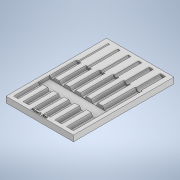
# Autodesk Inventor part: punchTray
Saved by Autodesk Inventor 2020.2 (Build 242310000, 310)
## iProperties
Created: 2019-12-07
Part Number: punchTray
Material: Generic
Document SubType Name: Modeling
Designer: robst
Density: 1 g/cm^3
Appearance: Default
Author: robst
Autodesk Inventor part; units mm, degrees
(part 1 of 2)
ref_plane "YZ Plane" through (0, 0, 0) normal (1, 0, 0) x (0, 1, 0)
ref_plane "XZ Plane" through (0, 0, 0) normal (0, 1, 0) x (-1, 0, 0)
ref_plane "XY Plane" through (0, 0, 0) normal (0, 0, 1) x (1, 0, 0)
sketch "Sketch3" plane through (0, 0, 0) normal (0, 0, 1) x (1, 0, 0)
  line L0 (-56.4324, -4.8895) -> (56.4324, -4.8895)
  line L1 (56.4324, -4.8895) -> (56.4324, 4.8895)
  line L2 (56.4324, 4.8895) -> (-56.4324, 4.8895)
  line L3 (-56.4324, 4.8895) -> (-56.4324, -4.8895)
  line L4 (-56.4324, -4.8895) -> (56.4324, 4.8895) construction
  line L5 (56.4324, -4.8895) -> (-56.4324, 4.8895) construction
  line L6 (50.0824, 4.8895) -> (47.1861, -0.127)
  line L7 (47.1861, -0.127) -> (41.3935, -0.127)
  line L8 (41.3935, -0.127) -> (38.4972, 4.8895)
  line L9 (38.4972, 4.8895) -> (41.3935, 9.906)
  line L10 (41.3935, 9.906) -> (47.1861, 9.906)
  line L11 (47.1861, 9.906) -> (50.0824, 4.8895)
  line L12 (30.5597, 4.8895) -> (27.6635, -0.127)
  line L13 (27.6635, -0.127) -> (21.8709, -0.127)
  line L14 (21.8709, -0.127) -> (18.9746, 4.8895)
  line L15 (18.9746, 4.8895) -> (21.8709, 9.906)
  line L16 (21.8709, 9.906) -> (27.6635, 9.906)
  line L17 (27.6635, 9.906) -> (30.5597, 4.8895)
  line L18 (0, 0) -> (0, 4.8895) construction
  line L19 (11.0371, 4.8895) -> (8.5808, 0.635)
  line L20 (8.5808, 0.635) -> (3.6681, 0.635)
  line L21 (3.6681, 0.635) -> (1.2118, 4.8895)
  line L22 (1.2118, 4.8895) -> (3.6681, 9.144)
  line L23 (3.6681, 9.144) -> (8.5808, 9.144)
  line L24 (8.5808, 9.144) -> (11.0371, 4.8895)
  line L25 (-6.7257, 4.8895) -> (-9.182, 0.635)
  line L26 (-9.182, 0.635) -> (-14.0947, 0.635)
  line L27 (-14.0947, 0.635) -> (-16.5511, 4.8895)
  line L28 (-16.5511, 4.8895) -> (-14.0947, 9.144)
  line L29 (-14.0947, 9.144) -> (-9.182, 9.144)
  line L30 (-9.182, 9.144) -> (-6.7257, 4.8895)
  line L31 (-24.4886, 4.8895) -> (-26.9229, 0.6731)
  line L32 (-26.9229, 0.6731) -> (-31.7916, 0.6731)
  line L33 (-31.7916, 0.6731) -> (-34.2259, 4.8895)
  line L34 (-34.2259, 4.8895) -> (-31.7916, 9.1059)
  line L35 (-31.7916, 9.1059) -> (-26.9229, 9.1059)
  line L36 (-26.9229, 9.1059) -> (-24.4886, 4.8895)
  line L37 (-42.1634, 4.8895) -> (-44.1432, 1.4605)
  line L38 (-44.1432, 1.4605) -> (-48.1026, 1.4605)
  line L39 (-48.1026, 1.4605) -> (-50.0824, 4.8895)
  line L40 (-50.0824, 4.8895) -> (-48.1026, 8.3185)
  line L41 (-48.1026, 8.3185) -> (-44.1432, 8.3185)
  line L42 (-44.1432, 8.3185) -> (-42.1634, 4.8895)
  point P0 (44.2898, 4.8895)
  point P1 (24.7672, 4.8895)
  point P2 (38.4972, 4.8895)
  point P3 (18.9746, 4.8895)
  point P4 (6.1245, 4.8895)
  point P5 (-11.6384, 4.8895)
  point P6 (-29.3572, 4.8895)
  point P7 (-46.1229, 4.8895)
  point P8 (1.2118, 4.8895)
  point P9 (-16.5511, 4.8895)
  point P10 (-34.2259, 4.8895)
  point P11 (-50.0824, 4.8895)
  dimension "d7" = 10.033
  dimension "d8" = 10.033
  dimension "d13" = 6.35
  dimension "d14" = 7.9375
  dimension "d15" = 8.509
  dimension "d16" = 7.9375
  dimension "d17" = 8.509
  dimension "d18" = 7.9375
  dimension "d19" = 8.4328
  dimension "d20" = 7.9375
  dimension "d21" = 7.9375
  dimension "d22" = 6.858
  dimension "d23" = 6.35
  dimension "d24" = 4.7625
  constraints: 84 end point, 2 horizontal, 2 midpoint, 1 parallel, 1 perpendicular, 94 other
  measures "d7" distance between parallel lines of L7 L10
  measures "d8" distance between parallel lines of L13 L16
  measures "d13" distance of L6.start L1.end
  measures "d14" distance of L8.end L12.start
  measures "d15" distance between parallel lines of L20 L23
  measures "d16" distance of L14.end L19.start
  measures "d17" distance between parallel lines of L26 L29
  measures "d18" distance of L21.end L25.start
  measures "d19" distance between parallel lines of L32 L35
  measures "d20" distance of L27.end L31.start
  measures "d21" distance of L33.end L37.start
  measures "d22" distance between parallel lines of L38 L41
  measures "d23" distance from line of L39.end L3
  measures "d24" distance between parallel lines of L0 L7
extrude "Extrusion3" add sketch "Sketch3" against normal blind 155.575 contours L3 L2 L39 L38 L37 L33 L32 L31 L27 L26 L25 L21 L20 L19 L14 L13 L12 L8 L7 L6 L1 L0
sketch "Sketch4" plane through (0, 0, 0) normal (0, 0, 1) x (1, 0, 0)
  line L0 (56.4324, -4.8895) -> (-56.4324, -4.8895) projected
  line L1 (56.4324, 4.8895) -> (56.4324, -4.8895) projected
  line L2 (-56.4324, -4.8895) -> (56.4324, -4.8895)
  line L3 (56.4324, -4.8895) -> (56.4324, 4.8895)
  line L4 (56.4324, 4.8895) -> (-56.4324, 4.8895)
  line L5 (-56.4324, 4.8895) -> (-56.4324, -4.8895)
  point P0 (0, 0)
  constraints: 8 end point, 2 parallel, 1 horizontal, 1 perpendicular
extrude "Extrusion4" add sketch "Sketch4" along normal blind 6.35
sketch "Sketch6" plane through (0, 0, -155.575) normal (0, 0, -1) x (-1, 0, 0)
  line L0 (-41.3935, -0.127) -> (-47.1861, -0.127) construction
  line L1 (-44.2898, -0.127) -> (-44.2898, 4.8895) construction
  line L2 (-56.4324, 4.8895) -> (56.4324, 4.8895) construction
  arc A0 (-48.5125, 4.8895) -> (-40.067, 4.8895) centre (-44.2898, 4.8895) ccw
  line L3 (-38.4972, 4.8895) -> (-41.3935, -0.127)
  line L4 (-41.3935, -0.127) -> (-47.1861, -0.127)
  line L5 (-47.1861, -0.127) -> (-50.0824, 4.8895)
  line L6 (-50.0824, 4.8895) -> (-48.5125, 4.8895)
  line L7 (-38.4972, 4.8895) -> (-40.067, 4.8895)
  point P0 (0, 0)
  dimension "d31" = 8.4455
  constraints: 12 end point, 3 point on line, 2 coincident, 2 point on circle, 1 centre point, 1 midpoint, 1 vertical, 6 other
  measures "d31" diameter of A0
extrude "5_16_punch" add sketch "Sketch6" against normal blind 40.64
sketch "Sketch7" plane through (0, 0, -155.575) normal (0, 0, -1) x (-1, 0, 0)
  line L0 (-30.5597, 4.8895) -> (-18.9746, 4.8895) projected
  line L1 (-18.9746, 4.8895) -> (-21.8709, -0.127)
  line L2 (-21.8709, -0.127) -> (-27.6635, -0.127)
  line L3 (-27.6635, -0.127) -> (-30.5597, 4.8895)
  arc A0 (-28.1962, 4.8895) -> (-21.3382, 4.8895) centre (-24.7672, 4.8895) ccw
  line L4 (-30.5597, 4.8895) -> (-28.1962, 4.8895)
  line L5 (-11.0371, 4.8895) -> (-18.9746, 4.8895) projected
  line L6 (-18.9746, 4.8895) -> (-21.3382, 4.8895)
  point P0 (0, 0)
  point P1 (-30.5597, 4.8895)
  dimension "d34" = 6.858
  constraints: 10 end point, 2 point on circle, 2 point on line, 1 centre point, 1 coincident, 1 midpoint, 6 other
  measures "d34" diameter of A0
extrude "1_4_punch" add sketch "Sketch7" against normal blind 40.64 contours L0 A0 L1 L2 L3
sketch "Sketch8" plane through (0, 0, -155.575) normal (0, 0, -1) x (-1, 0, 0)
  line L0 (-11.0371, 4.8895) -> (-1.2118, 4.8895) projected
  line L1 (-1.2118, 4.8895) -> (-3.6681, 0.635)
  line L2 (-3.6681, 0.635) -> (-8.5808, 0.635)
  line L3 (-8.5808, 0.635) -> (-11.0371, 4.8895)
  arc A0 (-8.7597, 4.8895) -> (-3.4892, 4.8895) centre (-6.1245, 4.8895) ccw
  line L4 (-11.0371, 4.8895) -> (-8.5808, 0.635) projected
  line L5 (-11.0371, 4.8895) -> (-8.7597, 4.8895)
  line L6 (-1.2118, 4.8895) -> (-3.4892, 4.8895)
  point P0 (0, 0)
  point P1 (-11.0371, 4.8895)
  dimension "d37" = 5.2705
  constraints: 10 end point, 2 point on circle, 2 point on line, 1 centre point, 1 coincident, 1 midpoint, 6 other
  measures "d37" diameter of A0
extrude "3_16_punch" add sketch "Sketch8" against normal blind 40.64 contours L0 A0 L1 L2 L3
sketch "Sketch9" plane through (0, 0, -155.575) normal (0, 0, -1) x (-1, 0, 0)
  line L0 (14.0947, 0.635) -> (9.182, 0.635) construction
  line L1 (11.6384, 0.635) -> (11.6384, 4.8895) construction
  line L2 (-56.4324, 4.8895) -> (56.4324, 4.8895) construction
  line L3 (16.5511, 4.8895) -> (14.0947, 0.635) projected
  line L4 (16.5511, 4.8895) -> (14.0947, 0.635)
  line L5 (14.0947, 0.635) -> (9.182, 0.635)
  line L6 (9.182, 0.635) -> (6.7257, 4.8895)
  arc A0 (9.4, 4.8895) -> (13.8768, 4.8895) centre (11.6384, 4.8895) ccw
  line L7 (9.182, 0.635) -> (6.7257, 4.8895) projected
  line L8 (6.7257, 4.8895) -> (9.4, 4.8895)
  line L9 (24.4886, 4.8895) -> (16.5511, 4.8895) projected
  line L10 (16.5511, 4.8895) -> (13.8768, 4.8895)
  point P0 (0, 0)
  point P1 (14.0947, 0.635)
  dimension "d40" = 4.4768
  constraints: 12 end point, 3 point on line, 2 coincident, 2 point on circle, 1 centre point, 1 midpoint, 1 vertical, 6 other
  measures "d40" diameter of A0
extrude "5_32_punch" add sketch "Sketch9" against normal blind 45.72
sketch "Sketch11" plane through (0, 0, -155.575) normal (0, 0, -1) x (-1, 0, 0)
  line L0 (24.4886, 4.8895) -> (34.2259, 4.8895) projected
  line L1 (31.7916, 0.6731) -> (34.2259, 4.8895) projected
  line L2 (34.2259, 4.8895) -> (31.7916, 0.6731)
  line L3 (31.7916, 0.6731) -> (26.9229, 0.6731)
  line L4 (26.9229, 0.6731) -> (24.4886, 4.8895)
  arc A0 (27.5157, 4.8895) -> (31.1987, 4.8895) centre (29.3572, 4.8895) ccw
  line L5 (24.4886, 4.8895) -> (26.9229, 0.6731) projected
  line L6 (24.4886, 4.8895) -> (27.5157, 4.8895)
  line L7 (34.2259, 4.8895) -> (31.1987, 4.8895)
  point P0 (0, 0)
  point P1 (31.7916, 0.6731)
  point P2 (24.4886, 4.8895)
  dimension "d44" = 3.683
  constraints: 10 end point, 2 point on circle, 2 point on line, 1 centre point, 1 coincident, 1 midpoint, 6 other
  measures "d44" diameter of A0
extrude "1_8_punch" add sketch "Sketch11" against normal blind 50.8 contours L0 A0 L1 L3 L4
sketch "Sketch12" plane through (0, 0, -155.575) normal (0, 0, -1) x (-1, 0, 0)
  line L0 (44.1432, 1.4605) -> (48.1026, 1.4605) construction
  line L1 (46.1229, 1.4605) -> (46.1229, 4.8895) construction
  line L2 (-56.4324, 4.8895) -> (56.4324, 4.8895) construction
  line L3 (48.1026, 1.4605) -> (50.0824, 4.8895) projected
  line L4 (50.0824, 4.8895) -> (48.1026, 1.4605)
  line L5 (48.1026, 1.4605) -> (44.1432, 1.4605)
  line L6 (44.1432, 1.4605) -> (42.1634, 4.8895)
  arc A0 (45.0751, 4.8895) -> (47.1706, 4.8895) centre (46.1229, 4.8895) ccw
  line L7 (42.1634, 4.8895) -> (31.1987, 4.8895) projected
  line L8 (42.1634, 4.8895) -> (45.0751, 4.8895)
  line L9 (50.0824, 4.8895) -> (47.1706, 4.8895)
  point P0 (0, 0)
  dimension "d47" = 2.0955
  constraints: 12 end point, 3 point on line, 2 coincident, 2 point on circle, 1 centre point, 1 midpoint, 1 vertical, 6 other
  measures "d47" diameter of A0
extrude "1_16_punch" add sketch "Sketch12" against normal blind 50.8
sketch "Sketch5" plane through (0, 0, -155.575) normal (0, 0, -1) x (-1, 0, 0)
  line L0 (-56.4324, 4.8895) -> (-56.4324, -4.8895) projected
  line L1 (56.4324, 4.8895) -> (50.0824, 4.8895) projected
  line L2 (-56.4324, -4.8895) -> (56.4324, -4.8895)
  line L3 (56.4324, -4.8895) -> (56.4324, 4.8895)
  line L4 (56.4324, 4.8895) -> (-56.4324, 4.8895)
  line L5 (-56.4324, 4.8895) -> (-56.4324, -4.8895)
  point P0 (0, 0)
  point P1 (-56.4324, 4.8895)
  constraints: 8 end point, 2 parallel, 1 horizontal, 1 perpendicular
extrude "Extrusion5" add sketch "Sketch5" along normal blind 6.35
sketch "Sketch13" plane through (-56.4324, 4.8895, 6.35) normal (0, 1, 0) x (1, 0, 0)
  line L0 (6.35, 6.35) -> (6.35, 111.125) projected
  line L1 (106.5147, 6.35) -> (106.5147, 121.285) projected
  line L2 (6.35, 47.625) -> (106.5147, 47.625)
  line L3 (106.5147, 47.625) -> (106.5147, 66.675)
  line L4 (106.5147, 66.675) -> (6.35, 66.675)
  line L5 (6.35, 66.675) -> (6.35, 47.625)
  line L6 (6.35, 57.15) -> (106.5147, 57.15) construction
  line L7 (14.2689, 6.35) -> (6.35, 6.35) construction
  point P0 (56.4324, 6.35)
  point P1 (6.35, 66.675)
  point P2 (106.5147, 47.625)
  dimension "d50" = 19.05
  dimension "d51" = 50.8
  constraints: 10 end point, 2 midpoint, 2 parallel, 2 point on line, 1 horizontal, 1 perpendicular
  measures "d50" distance between parallel lines of L4 L2
  measures "d51" distance between parallel lines of L6 L7
extrude "Extrusion12" cut sketch "Sketch13" against normal blind 5.08
sketch "Sketch14" plane through (-56.4324, 4.8895, 6.35) normal (0, 1, 0) x (1, 0, 0)
  line L0 (0, 168.275) -> (0, 0) construction
  line L1 (0, 3.175) -> (104.9272, 3.175) construction
  line L2 (0, 0) -> (112.8647, 0) construction
  spline S0 degree 2 poles (42.5851, 3.879) (42.5851, 3.6134) (42.4153, 3.1318) (42.2578, 2.9712) knots 0 0 0 1 2 2 2
  spline S1 degree 2 poles (42.2578, 2.9712) (42.1621, 2.8693) (41.9274, 2.7026) (41.7885, 2.6439) knots 0 0 0 1 2 2 2
  spline S2 degree 2 poles (41.7885, 2.6439) (41.6465, 2.5853) (41.3161, 2.5174) (41.1123, 2.5174) knots 0 0 0 1 2 2 2
  line L3 (41.1123, 2.5174) -> (40.6122, 2.5174)
  line L4 (40.6122, 2.5174) -> (40.6122, 1.27)
  line L5 (40.6122, 1.27) -> (39.655, 1.27)
  line L6 (39.655, 1.27) -> (39.655, 5.08)
  line L7 (39.655, 5.08) -> (41.1339, 5.08)
  spline S3 degree 2 poles (41.1339, 5.08) (41.4612, 5.08) (41.9398, 4.9596) (42.1343, 4.8299) knots 0 0 0 1 2 2 2
  spline S4 degree 2 poles (42.1343, 4.8299) (42.3504, 4.6848) (42.5851, 4.2093) (42.5851, 3.879) knots 0 0 0 1 2 2 2
  spline S5 degree 2 poles (41.6033, 3.8543) (41.6033, 4.0179) (41.4489, 4.2495) (41.3439, 4.2927) knots 0 0 0 1 2 2 2
  spline S6 degree 2 poles (41.3439, 4.2927) (41.208, 4.3513) (40.961, 4.3699) (40.748, 4.3699) knots 0 0 0 1 2 2 2
  line L8 (40.748, 4.3699) -> (40.6122, 4.3699)
  line L9 (40.6122, 4.3699) -> (40.6122, 3.2275)
  line L10 (40.6122, 3.2275) -> (40.6801, 3.2275)
  spline S7 degree 2 poles (40.6801, 3.2275) (40.8128, 3.2275) (41.0537, 3.2337) (41.1432, 3.2491) knots 0 0 0 1 2 2 2
  spline S8 degree 2 poles (41.1432, 3.2491) (41.2204, 3.2615) (41.3902, 3.3356) (41.4365, 3.3819) knots 0 0 0 1 2 2 2
  spline S9 degree 2 poles (41.4365, 3.3819) (41.5353, 3.4745) (41.6033, 3.6814) (41.6033, 3.8543) knots 0 0 0 1 2 2 2
  line L11 (45.7127, 1.27) -> (44.8174, 1.27)
  line L12 (44.8174, 1.27) -> (44.8174, 1.588)
  spline S10 degree 2 poles (44.8174, 1.588) (44.5858, 1.3935) (44.1968, 1.1897) (43.9282, 1.1897) knots 0 0 0 1 2 2 2
  spline S11 degree 2 poles (43.9282, 1.1897) (43.5021, 1.1897) (43.0235, 1.73) (43.0235, 2.2734) knots 0 0 0 1 2 2 2
  line L13 (43.0235, 2.2734) -> (43.0235, 4.1445)
  line L14 (43.0235, 4.1445) -> (43.9251, 4.1445)
  line L15 (43.9251, 4.1445) -> (43.9251, 2.718)
  spline S12 degree 2 poles (43.9251, 2.718) (43.9251, 2.4957) (43.9467, 2.2117) (43.9899, 2.116) knots 0 0 0 1 2 2 2
  spline S13 degree 2 poles (43.9899, 2.116) (44.0331, 2.0264) (44.2029, 1.9338) (44.3573, 1.9338) knots 0 0 0 1 2 2 2
  spline S14 degree 2 poles (44.3573, 1.9338) (44.4499, 1.9338) (44.7093, 2.0264) (44.8174, 2.1067) knots 0 0 0 1 2 2 2
  line L16 (44.8174, 2.1067) -> (44.8174, 4.1445)
  line L17 (44.8174, 4.1445) -> (45.7127, 4.1445)
  line L18 (45.7127, 4.1445) -> (45.7127, 1.27)
  line L19 (49.0874, 1.27) -> (48.1858, 1.27)
  line L20 (48.1858, 1.27) -> (48.1858, 2.6933)
  spline S15 degree 2 poles (48.1858, 2.6933) (48.1858, 2.8693) (48.1581, 3.2151) (48.121, 3.2954) knots 0 0 0 1 2 2 2
  spline S16 degree 2 poles (48.121, 3.2954) (48.0747, 3.3942) (47.9018, 3.4776) (47.7536, 3.4776) knots 0 0 0 1 2 2 2
  spline S17 degree 2 poles (47.7536, 3.4776) (47.6455, 3.4776) (47.4201, 3.3942) (47.2936, 3.3047) knots 0 0 0 1 2 2 2
  line L21 (47.2936, 3.3047) -> (47.2936, 1.27)
  line L22 (47.2936, 1.27) -> (46.3982, 1.27)
  line L23 (46.3982, 1.27) -> (46.3982, 4.1445)
  line L24 (46.3982, 4.1445) -> (47.2936, 4.1445)
  line L25 (47.2936, 4.1445) -> (47.2936, 3.8265)
  spline S18 degree 2 poles (47.2936, 3.8265) (47.5128, 4.0117) (47.9296, 4.2217) (48.1828, 4.2217) knots 0 0 0 1 2 2 2
  spline S19 degree 2 poles (48.1828, 4.2217) (48.6212, 4.2217) (49.0874, 3.6659) (49.0874, 3.141) knots 0 0 0 1 2 2 2
  line L26 (49.0874, 3.141) -> (49.0874, 1.27)
  spline S20 degree 2 poles (51.1591, 1.1928) (50.8041, 1.1928) (50.2143, 1.3719) (49.9951, 1.5571) knots 0 0 0 1 2 2 2
  spline S21 degree 2 poles (49.9951, 1.5571) (49.7821, 1.7455) (49.5413, 2.3105) (49.5413, 2.6933) knots 0 0 0 1 2 2 2
  spline S22 degree 2 poles (49.5413, 2.6933) (49.5413, 3.1071) (49.8006, 3.6844) (50.026, 3.8697) knots 0 0 0 1 2 2 2
  spline S23 degree 2 poles (50.026, 3.8697) (50.239, 4.0488) (50.8195, 4.2217) (51.1344, 4.2217) knots 0 0 0 1 2 2 2
  spline S24 degree 2 poles (51.1344, 4.2217) (51.3722, 4.2217) (51.8476, 4.1105) (52.0885, 3.9901) knots 0 0 0 1 2 2 2
  line L27 (52.0885, 3.9901) -> (52.0885, 3.2244)
  line L28 (52.0885, 3.2244) -> (51.9742, 3.2244)
  spline S25 degree 2 poles (51.9742, 3.2244) (51.9187, 3.2769) (51.7643, 3.4004) (51.6717, 3.4498) knots 0 0 0 1 2 2 2
  spline S26 degree 2 poles (51.6717, 3.4498) (51.5729, 3.5054) (51.3289, 3.5795) (51.1777, 3.5795) knots 0 0 0 1 2 2 2
  spline S27 degree 2 poles (51.1777, 3.5795) (50.8349, 3.5795) (50.4583, 3.1009) (50.4583, 2.6933) knots 0 0 0 1 2 2 2
  spline S28 degree 2 poles (50.4583, 2.6933) (50.4583, 2.2611) (50.8596, 1.835) (51.1931, 1.835) knots 0 0 0 1 2 2 2
  spline S29 degree 2 poles (51.1931, 1.835) (51.3629, 1.835) (51.6161, 1.9122) (51.7087, 1.9678) knots 0 0 0 1 2 2 2
  spline S30 degree 2 poles (51.7087, 1.9678) (51.7982, 2.0203) (51.9279, 2.1376) (51.9742, 2.1839) knots 0 0 0 1 2 2 2
  line L29 (51.9742, 2.1839) -> (52.0885, 2.1839)
  line L30 (52.0885, 2.1839) -> (52.0885, 1.4151)
  spline S31 degree 2 poles (52.0885, 1.4151) (52.0113, 1.3812) (51.8106, 1.2947) (51.7056, 1.2669) knots 0 0 0 1 2 2 2
  spline S32 degree 2 poles (51.7056, 1.2669) (51.5759, 1.2299) (51.3475, 1.1928) (51.1591, 1.1928) knots 0 0 0 1 2 2 2
  line L31 (55.2038, 1.27) -> (54.3022, 1.27)
  line L32 (54.3022, 1.27) -> (54.3022, 2.6933)
  spline S33 degree 2 poles (54.3022, 2.6933) (54.3022, 2.8693) (54.2744, 3.2151) (54.2374, 3.2954) knots 0 0 0 1 2 2 2
  spline S34 degree 2 poles (54.2374, 3.2954) (54.1911, 3.3942) (54.0182, 3.4776) (53.87, 3.4776) knots 0 0 0 1 2 2 2
  spline S35 degree 2 poles (53.87, 3.4776) (53.7619, 3.4776) (53.5365, 3.3942) (53.4099, 3.3047) knots 0 0 0 1 2 2 2
  line L33 (53.4099, 3.3047) -> (53.4099, 1.27)
  line L34 (53.4099, 1.27) -> (52.5145, 1.27)
  line L35 (52.5145, 1.27) -> (52.5145, 5.2498)
  line L36 (52.5145, 5.2498) -> (53.4099, 5.2498)
  line L37 (53.4099, 5.2498) -> (53.4099, 3.8265)
  spline S36 degree 2 poles (53.4099, 3.8265) (53.6291, 4.0117) (54.046, 4.2217) (54.2991, 4.2217) knots 0 0 0 1 2 2 2
  spline S37 degree 2 poles (54.2991, 4.2217) (54.7376, 4.2217) (55.2038, 3.6659) (55.2038, 3.141) knots 0 0 0 1 2 2 2
  line L38 (55.2038, 3.141) -> (55.2038, 1.27)
  spline S38 degree 2 poles (58.6309, 1.2021) (58.1925, 1.2021) (57.5318, 1.3719) (57.2477, 1.4954) knots 0 0 0 1 2 2 2
  line L39 (57.2477, 1.4954) -> (57.2477, 2.4031)
  line L40 (57.2477, 2.4031) -> (57.3342, 2.4031)
  spline S39 degree 2 poles (57.3342, 2.4031) (57.6213, 2.1592) (58.3098, 1.8968) (58.634, 1.8968) knots 0 0 0 1 2 2 2
  spline S40 degree 2 poles (58.634, 1.8968) (58.7174, 1.8968) (58.986, 1.9338) (59.0663, 1.9709) knots 0 0 0 1 2 2 2
  spline S41 degree 2 poles (59.0663, 1.9709) (59.1651, 2.0141) (59.304, 2.1716) (59.304, 2.2981) knots 0 0 0 1 2 2 2
  spline S42 degree 2 poles (59.304, 2.2981) (59.304, 2.4433) (59.0786, 2.6223) (58.9242, 2.6625) knots 0 0 0 1 2 2 2
  spline S43 degree 2 poles (58.9242, 2.6625) (58.7297, 2.715) (58.2882, 2.8045) (58.0937, 2.8724) knots 0 0 0 1 2 2 2
  spline S44 degree 2 poles (58.0937, 2.8724) (57.6522, 3.0268) (57.2693, 3.5548) (57.2693, 3.95) knots 0 0 0 1 2 2 2
  spline S45 degree 2 poles (57.2693, 3.95) (57.2693, 4.4841) (58.174, 5.1479) (58.8532, 5.1479) knots 0 0 0 1 2 2 2
  spline S46 degree 2 poles (58.8532, 5.1479) (59.1929, 5.1479) (59.8659, 5.009) (60.1315, 4.8917) knots 0 0 0 1 2 2 2
  line L41 (60.1315, 4.8917) -> (60.1315, 4.021)
  line L42 (60.1315, 4.021) -> (60.0481, 4.021)
  spline S47 degree 2 poles (60.0481, 4.021) (59.8351, 4.2031) (59.2237, 4.4532) (58.9026, 4.4532) knots 0 0 0 1 2 2 2
  spline S48 degree 2 poles (58.9026, 4.4532) (58.776, 4.4532) (58.5784, 4.4162) (58.4673, 4.3668) knots 0 0 0 1 2 2 2
  spline S49 degree 2 poles (58.4673, 4.3668) (58.3778, 4.3266) (58.2481, 4.1661) (58.2481, 4.0673) knots 0 0 0 1 2 2 2
  spline S50 degree 2 poles (58.2481, 4.0673) (58.2481, 3.9191) (58.4549, 3.7493) (58.7513, 3.6814) knots 0 0 0 1 2 2 2
  spline S51 degree 2 poles (58.7513, 3.6814) (58.9428, 3.6381) (59.2978, 3.5548) (59.5016, 3.4838) knots 0 0 0 1 2 2 2
  spline S52 degree 2 poles (59.5016, 3.4838) (59.8968, 3.3386) (60.2828, 2.857) (60.2828, 2.4618) knots 0 0 0 1 2 2 2
  spline S53 degree 2 poles (60.2828, 2.4618) (60.2828, 1.8937) (59.3905, 1.2021) (58.6309, 1.2021) knots 0 0 0 1 2 2 2
  spline S54 degree 2 poles (62.1939, 1.1928) (61.3788, 1.1928) (60.5112, 1.9709) (60.5112, 2.6903) knots 0 0 0 1 2 2 2
  spline S55 degree 2 poles (60.5112, 2.6903) (60.5112, 3.3942) (61.3202, 4.234) (62.0488, 4.234) knots 0 0 0 1 2 2 2
  spline S56 degree 2 poles (62.0488, 4.234) (62.7065, 4.234) (63.3734, 3.5208) (63.3734, 2.8601) knots 0 0 0 1 2 2 2
  line L43 (63.3734, 2.8601) -> (63.3734, 2.5359)
  line L44 (63.3734, 2.5359) -> (61.4066, 2.5359)
  spline S57 degree 2 poles (61.4066, 2.5359) (61.419, 2.3352) (61.5641, 2.0697) (61.6814, 1.9894) knots 0 0 0 1 2 2 2
  spline S58 degree 2 poles (61.6814, 1.9894) (61.7956, 1.9091) (62.1044, 1.8412) (62.2866, 1.8412) knots 0 0 0 1 2 2 2
  spline S59 degree 2 poles (62.2866, 1.8412) (62.4409, 1.8412) (62.7435, 1.9091) (62.8701, 1.9678) knots 0 0 0 1 2 2 2
  spline S60 degree 2 poles (62.8701, 1.9678) (62.9812, 2.0141) (63.1665, 2.1283) (63.2252, 2.1716) knots 0 0 0 1 2 2 2
  line L45 (63.2252, 2.1716) -> (63.3209, 2.1716)
  line L46 (63.3209, 2.1716) -> (63.3209, 1.4306)
  spline S61 degree 2 poles (63.3209, 1.4306) (63.2097, 1.3873) (63.0306, 1.3132) (62.8701, 1.2762) knots 0 0 0 1 2 2 2
  spline S62 degree 2 poles (62.8701, 1.2762) (62.725, 1.236) (62.4162, 1.1928) (62.1939, 1.1928) knots 0 0 0 1 2 2 2
  spline S63 degree 2 poles (62.4903, 3.0762) (62.4842, 3.3603) (62.2341, 3.6597) (61.9778, 3.6597) knots 0 0 0 1 2 2 2
  spline S64 degree 2 poles (61.9778, 3.6597) (61.7154, 3.6597) (61.419, 3.3448) (61.4035, 3.0762) knots 0 0 0 1 2 2 2
  line L47 (61.4035, 3.0762) -> (62.4903, 3.0762)
  spline S65 degree 2 poles (64.9326, 1.2144) (64.3861, 1.2144) (63.8859, 1.6652) (63.8859, 2.1777) knots 0 0 0 1 2 2 2
  line L48 (63.8859, 2.1777) -> (63.8859, 3.5208)
  line L49 (63.8859, 3.5208) -> (63.5432, 3.5208)
  line L50 (63.5432, 3.5208) -> (63.5432, 4.1445)
  line L51 (63.5432, 4.1445) -> (63.8859, 4.1445)
  line L52 (63.8859, 4.1445) -> (63.8859, 4.9658)
  line L53 (63.8859, 4.9658) -> (64.7813, 4.9658)
  line L54 (64.7813, 4.9658) -> (64.7813, 4.1445)
  line L55 (64.7813, 4.1445) -> (65.6458, 4.1445)
  line L56 (65.6458, 4.1445) -> (65.6458, 3.5208)
  line L57 (65.6458, 3.5208) -> (64.7813, 3.5208)
  line L58 (64.7813, 3.5208) -> (64.7813, 2.4988)
  spline S66 degree 2 poles (64.7813, 2.4988) (64.7813, 2.3475) (64.7874, 2.1222) (64.8245, 2.0326) knots 0 0 0 1 2 2 2
  spline S67 degree 2 poles (64.8245, 2.0326) (64.8615, 1.9431) (65.0437, 1.8381) (65.2166, 1.8381) knots 0 0 0 1 2 2 2
  spline S68 degree 2 poles (65.2166, 1.8381) (65.2907, 1.8381) (65.5223, 1.8999) (65.5686, 1.9246) knots 0 0 0 1 2 2 2
  line L59 (65.5686, 1.9246) -> (65.6458, 1.9246)
  line L60 (65.6458, 1.9246) -> (65.6458, 1.2947)
  spline S69 degree 2 poles (65.6458, 1.2947) (65.5007, 1.2576) (65.1734, 1.2144) (64.9326, 1.2144) knots 0 0 0 1 2 2 2
  point P0 (56.4324, 6.35)
  dimension "d54" = 3.175
  constraints: 2 end point, 1 horizontal, 1 parallel, 1 point on line
  measures "d54" distance between parallel lines of L1 L2
extrude "Extrusion13" cut sketch "Sketch14" against normal blind 3.175
sketch "Sketch15" plane through (-56.4324, -4.8895, 6.35) normal (0, -1, 0) x (1, 0, 0)
  line L0 (112.8647, -168.275) -> (112.8647, 0) construction
  line L1 (112.8647, -84.1375) -> (0, -84.1375) construction
  line L2 (0, -168.275) -> (0, 0) construction
  spline S0 degree 2 poles (77.0158, -94.2924) (77.0158, -93.4021) (77.7928, -92.0024) (78.3846, -91.6268) knots 0 0 0 1 2 2 2
  spline S1 degree 2 poles (78.3846, -91.6268) (78.8786, -91.3078) (80.0416, -91.1225) (80.6951, -91.1225) knots 0 0 0 1 2 2 2
  line L3 (80.6951, -91.1225) -> (82.6814, -91.1225)
  line L4 (82.6814, -91.1225) -> (82.6814, -97.4725)
  line L5 (82.6814, -97.4725) -> (80.7157, -97.4725)
  spline S2 degree 2 poles (80.7157, -97.4725) (80.0467, -97.4725) (78.8786, -97.3027) (78.364, -96.9734) knots 0 0 0 1 2 2 2
  spline S3 degree 2 poles (78.364, -96.9734) (77.7414, -96.572) (77.0158, -95.2135) (77.0158, -94.2924) knots 0 0 0 1 2 2 2
  spline S4 degree 2 poles (78.6522, -94.3026) (78.6522, -94.9304) (79.0845, -95.8258) (79.527, -96.078) knots 0 0 0 1 2 2 2
  spline S5 degree 2 poles (79.527, -96.078) (79.8512, -96.2529) (80.5613, -96.289) (81.0553, -96.289) knots 0 0 0 1 2 2 2
  line L6 (81.0553, -96.289) -> (81.0862, -96.289)
  line L7 (81.0862, -96.289) -> (81.0862, -92.3112)
  line L8 (81.0862, -92.3112) -> (81.0553, -92.3112)
  spline S6 degree 2 poles (81.0553, -92.3112) (80.5202, -92.3112) (79.7843, -92.3472) (79.4498, -92.5582) knots 0 0 0 1 2 2 2
  spline S7 degree 2 poles (79.4498, -92.5582) (79.0587, -92.8052) (78.6522, -93.6749) (78.6522, -94.3026) knots 0 0 0 1 2 2 2
  spline S8 degree 2 poles (73.7019, -90.9939) (75.0604, -90.9939) (76.5064, -92.2906) (76.5064, -93.4896) knots 0 0 0 1 2 2 2
  spline S9 degree 2 poles (76.5064, -93.4896) (76.5064, -94.6629) (75.1582, -96.0625) (73.9437, -96.0625) knots 0 0 0 1 2 2 2
  spline S10 degree 2 poles (73.9437, -96.0625) (72.8477, -96.0625) (71.7362, -94.8738) (71.7362, -93.7726) knots 0 0 0 1 2 2 2
  line L9 (71.7362, -93.7726) -> (71.7362, -93.2323)
  line L10 (71.7362, -93.2323) -> (75.0141, -93.2323)
  spline S11 degree 2 poles (75.0141, -93.2323) (74.9935, -92.8978) (74.7516, -92.4553) (74.5561, -92.3215) knots 0 0 0 1 2 2 2
  spline S12 degree 2 poles (74.5561, -92.3215) (74.3657, -92.1877) (73.8511, -92.0745) (73.5475, -92.0745) knots 0 0 0 1 2 2 2
  spline S13 degree 2 poles (73.5475, -92.0745) (73.2902, -92.0745) (72.7859, -92.1877) (72.5749, -92.2855) knots 0 0 0 1 2 2 2
  spline S14 degree 2 poles (72.5749, -92.2855) (72.3897, -92.3627) (72.0809, -92.5531) (71.9832, -92.6251) knots 0 0 0 1 2 2 2
  line L11 (71.9832, -92.6251) -> (71.8236, -92.6251)
  line L12 (71.8236, -92.6251) -> (71.8236, -91.3901)
  spline S15 degree 2 poles (71.8236, -91.3901) (72.0089, -91.318) (72.3074, -91.1945) (72.5749, -91.1328) knots 0 0 0 1 2 2 2
  spline S16 degree 2 poles (72.5749, -91.1328) (72.8168, -91.0659) (73.3314, -90.9939) (73.7019, -90.9939) knots 0 0 0 1 2 2 2
  spline S17 degree 2 poles (73.2079, -94.1328) (73.2182, -94.6063) (73.635, -95.1054) (74.0621, -95.1054) knots 0 0 0 1 2 2 2
  spline S18 degree 2 poles (74.0621, -95.1054) (74.4995, -95.1054) (74.9935, -94.5805) (75.0192, -94.1328) knots 0 0 0 1 2 2 2
  line L13 (75.0192, -94.1328) -> (73.2079, -94.1328)
  spline S19 degree 2 poles (69.5131, -90.9939) (70.038, -90.9939) (70.9797, -91.2254) (71.2885, -91.3798) knots 0 0 0 1 2 2 2
  line L14 (71.2885, -91.3798) -> (71.2885, -92.6405)
  line L15 (71.2885, -92.6405) -> (71.165, -92.6405)
  spline S20 degree 2 poles (71.165, -92.6405) (71.0569, -92.5582) (70.7842, -92.3627) (70.5423, -92.2546) knots 0 0 0 1 2 2 2
  spline S21 degree 2 poles (70.5423, -92.2546) (70.3313, -92.1568) (69.8116, -92.0179) (69.5029, -92.0179) knots 0 0 0 1 2 2 2
  spline S22 degree 2 poles (69.5029, -92.0179) (69.189, -92.0179) (68.7052, -92.2134) (68.7052, -92.4244) knots 0 0 0 1 2 2 2
  spline S23 degree 2 poles (68.7052, -92.4244) (68.7052, -92.5891) (68.9265, -92.764) (69.2456, -92.8361) knots 0 0 0 1 2 2 2
  spline S24 degree 2 poles (69.2456, -92.8361) (69.4154, -92.8824) (69.9351, -92.9802) (70.1358, -93.0419) knots 0 0 0 1 2 2 2
  spline S25 degree 2 poles (70.1358, -93.0419) (70.7018, -93.2169) (71.2679, -93.9013) (71.2679, -94.4622) knots 0 0 0 1 2 2 2
  spline S26 degree 2 poles (71.2679, -94.4622) (71.2679, -94.7812) (70.9746, -95.3473) (70.6864, -95.5685) knots 0 0 0 1 2 2 2
  spline S27 degree 2 poles (70.6864, -95.5685) (70.4034, -95.7847) (69.5646, -96.0419) (69.0346, -96.0419) knots 0 0 0 1 2 2 2
  spline S28 degree 2 poles (69.0346, -96.0419) (68.5303, -96.0419) (67.6864, -95.8413) (67.3982, -95.7023) knots 0 0 0 1 2 2 2
  line L16 (67.3982, -95.7023) -> (67.3982, -94.4879)
  line L17 (67.3982, -94.4879) -> (67.5166, -94.4879)
  spline S29 degree 2 poles (67.5166, -94.4879) (67.5937, -94.5496) (67.9282, -94.7503) (68.0826, -94.8224) knots 0 0 0 1 2 2 2
  spline S30 degree 2 poles (68.0826, -94.8224) (68.273, -94.9047) (68.7361, -95.0179) (68.978, -95.0179) knots 0 0 0 1 2 2 2
  spline S31 degree 2 poles (68.978, -95.0179) (69.3022, -95.0179) (69.7499, -94.7966) (69.7499, -94.6165) knots 0 0 0 1 2 2 2
  spline S32 degree 2 poles (69.7499, -94.6165) (69.7499, -94.4519) (69.5286, -94.2666) (69.1581, -94.174) knots 0 0 0 1 2 2 2
  spline S33 degree 2 poles (69.1581, -94.174) (68.9677, -94.1277) (68.4685, -94.0402) (68.237, -93.963) knots 0 0 0 1 2 2 2
  spline S34 degree 2 poles (68.237, -93.963) (67.7224, -93.7984) (67.1872, -93.1551) (67.1872, -92.6199) knots 0 0 0 1 2 2 2
  spline S35 degree 2 poles (67.1872, -92.6199) (67.1872, -92.2855) (67.5011, -91.6731) (67.7944, -91.4673) knots 0 0 0 1 2 2 2
  spline S36 degree 2 poles (67.7944, -91.4673) (68.098, -91.2409) (68.9317, -90.9939) (69.5131, -90.9939) knots 0 0 0 1 2 2 2
  line L18 (64.9848, -91.1225) -> (66.4771, -91.1225)
  line L19 (66.4771, -91.1225) -> (66.4771, -95.9133)
  line L20 (66.4771, -95.9133) -> (64.9848, -95.9133)
  line L21 (64.9848, -95.9133) -> (64.9848, -91.1225)
  line L22 (64.9385, -96.5977) -> (66.5183, -96.5977)
  line L23 (66.5183, -96.5977) -> (66.5183, -97.7607)
  line L24 (66.5183, -97.7607) -> (64.9385, -97.7607)
  line L25 (64.9385, -97.7607) -> (64.9385, -96.5977)
  spline S37 degree 2 poles (59.489, -91.6731) (59.489, -91.0093) (59.8749, -90.0779) (60.2043, -89.8206) knots 0 0 0 1 2 2 2
  spline S38 degree 2 poles (60.2043, -89.8206) (60.5388, -89.5582) (61.465, -89.3214) (62.0311, -89.3214) knots 0 0 0 1 2 2 2
  spline S39 degree 2 poles (62.0311, -89.3214) (62.5096, -89.3214) (63.369, -89.4449) (63.6829, -89.5273) knots 0 0 0 1 2 2 2
  line L26 (63.6829, -89.5273) -> (63.6829, -90.7263)
  line L27 (63.6829, -90.7263) -> (63.5079, -90.7263)
  spline S40 degree 2 poles (63.5079, -90.7263) (63.3999, -90.6851) (63.0963, -90.5822) (62.9419, -90.541) knots 0 0 0 1 2 2 2
  spline S41 degree 2 poles (62.9419, -90.541) (62.7566, -90.4947) (62.4067, -90.433) (62.2266, -90.433) knots 0 0 0 1 2 2 2
  spline S42 degree 2 poles (62.2266, -90.433) (61.8458, -90.433) (61.3415, -90.5873) (61.2129, -90.7314) knots 0 0 0 1 2 2 2
  spline S43 degree 2 poles (61.2129, -90.7314) (61.0842, -90.8806) (60.9813, -91.282) (60.9813, -91.5908) knots 0 0 0 1 2 2 2
  line L28 (60.9813, -91.5908) -> (60.9813, -91.6783)
  spline S44 degree 2 poles (60.9813, -91.6783) (61.2334, -91.457) (61.8921, -91.1894) (62.242, -91.1894) knots 0 0 0 1 2 2 2
  spline S45 degree 2 poles (62.242, -91.1894) (63.1734, -91.1894) (64.182, -92.3987) (64.182, -93.6388) knots 0 0 0 1 2 2 2
  spline S46 degree 2 poles (64.182, -93.6388) (64.182, -94.1997) (63.8733, -95.0951) (63.5954, -95.409) knots 0 0 0 1 2 2 2
  spline S47 degree 2 poles (63.5954, -95.409) (63.3278, -95.7126) (62.5817, -96.0419) (62.1751, -96.0419) knots 0 0 0 1 2 2 2
  spline S48 degree 2 poles (62.1751, -96.0419) (61.8098, -96.0419) (61.2283, -95.8567) (60.9916, -95.7023) knots 0 0 0 1 2 2 2
  line L29 (60.9916, -95.7023) -> (60.935, -95.9133)
  line L30 (60.935, -95.9133) -> (59.489, -95.9133)
  line L31 (59.489, -95.9133) -> (59.489, -91.6731)
  line L32 (60.9813, -92.6302) -> (60.9813, -94.8018)
  spline S49 degree 2 poles (60.9813, -94.8018) (61.0894, -94.8533) (61.4136, -94.9201) (61.5782, -94.9201) knots 0 0 0 1 2 2 2
  spline S50 degree 2 poles (61.5782, -94.9201) (62.1134, -94.9201) (62.6537, -94.2255) (62.6537, -93.6028) knots 0 0 0 1 2 2 2
  spline S51 degree 2 poles (62.6537, -93.6028) (62.6537, -93.2941) (62.5714, -92.8618) (62.4633, -92.6971) knots 0 0 0 1 2 2 2
  spline S52 degree 2 poles (62.4633, -92.6971) (62.3552, -92.5325) (62.0105, -92.3678) (61.7429, -92.3678) knots 0 0 0 1 2 2 2
  spline S53 degree 2 poles (61.7429, -92.3678) (61.5422, -92.3678) (61.1563, -92.5067) (60.9813, -92.6302) knots 0 0 0 1 2 2 2
  line L33 (53.8646, -91.1225) -> (55.3672, -91.1225)
  line L34 (55.3672, -91.1225) -> (55.3672, -93.4947)
  spline S54 degree 2 poles (55.3672, -93.4947) (55.3672, -93.7881) (55.4135, -94.3644) (55.4752, -94.4982) knots 0 0 0 1 2 2 2
  spline S55 degree 2 poles (55.4752, -94.4982) (55.5524, -94.6629) (55.8406, -94.8018) (56.0876, -94.8018) knots 0 0 0 1 2 2 2
  spline S56 degree 2 poles (56.0876, -94.8018) (56.2677, -94.8018) (56.6433, -94.6629) (56.8543, -94.5136) knots 0 0 0 1 2 2 2
  line L35 (56.8543, -94.5136) -> (56.8543, -91.1225)
  line L36 (56.8543, -91.1225) -> (58.3466, -91.1225)
  line L37 (58.3466, -91.1225) -> (58.3466, -95.9133)
  line L38 (58.3466, -95.9133) -> (56.8543, -95.9133)
  line L39 (56.8543, -95.9133) -> (56.8543, -95.3833)
  spline S57 degree 2 poles (56.8543, -95.3833) (56.489, -95.692) (55.7943, -96.0419) (55.3723, -96.0419) knots 0 0 0 1 2 2 2
  spline S58 degree 2 poles (55.3723, -96.0419) (54.6416, -96.0419) (53.8646, -95.1157) (53.8646, -94.2409) knots 0 0 0 1 2 2 2
  line L40 (53.8646, -94.2409) -> (53.8646, -91.1225)
  spline S59 degree 2 poles (50.3036, -90.9939) (51.6621, -90.9939) (53.1081, -92.2906) (53.1081, -93.4896) knots 0 0 0 1 2 2 2
  spline S60 degree 2 poles (53.1081, -93.4896) (53.1081, -94.6629) (51.7599, -96.0625) (50.5455, -96.0625) knots 0 0 0 1 2 2 2
  spline S61 degree 2 poles (50.5455, -96.0625) (49.4494, -96.0625) (48.3379, -94.8738) (48.3379, -93.7726) knots 0 0 0 1 2 2 2
  line L41 (48.3379, -93.7726) -> (48.3379, -93.2323)
  line L42 (48.3379, -93.2323) -> (51.6158, -93.2323)
  spline S62 degree 2 poles (51.6158, -93.2323) (51.5952, -92.8978) (51.3534, -92.4553) (51.1578, -92.3215) knots 0 0 0 1 2 2 2
  spline S63 degree 2 poles (51.1578, -92.3215) (50.9674, -92.1877) (50.4529, -92.0745) (50.1492, -92.0745) knots 0 0 0 1 2 2 2
  spline S64 degree 2 poles (50.1492, -92.0745) (49.892, -92.0745) (49.3877, -92.1877) (49.1767, -92.2855) knots 0 0 0 1 2 2 2
  spline S65 degree 2 poles (49.1767, -92.2855) (48.9914, -92.3627) (48.6827, -92.5531) (48.5849, -92.6251) knots 0 0 0 1 2 2 2
  line L43 (48.5849, -92.6251) -> (48.4254, -92.6251)
  line L44 (48.4254, -92.6251) -> (48.4254, -91.3901)
  spline S66 degree 2 poles (48.4254, -91.3901) (48.6106, -91.318) (48.9091, -91.1945) (49.1767, -91.1328) knots 0 0 0 1 2 2 2
  spline S67 degree 2 poles (49.1767, -91.1328) (49.4185, -91.0659) (49.9331, -90.9939) (50.3036, -90.9939) knots 0 0 0 1 2 2 2
  spline S68 degree 2 poles (49.8096, -94.1328) (49.8199, -94.6063) (50.2367, -95.1054) (50.6638, -95.1054) knots 0 0 0 1 2 2 2
  spline S69 degree 2 poles (50.6638, -95.1054) (51.1012, -95.1054) (51.5952, -94.5805) (51.621, -94.1328) knots 0 0 0 1 2 2 2
  line L45 (51.621, -94.1328) -> (49.8096, -94.1328)
  line L46 (43.2178, -91.1225) -> (44.7101, -91.1225)
  line L47 (44.7101, -91.1225) -> (44.7101, -91.6216)
  spline S70 degree 2 poles (44.7101, -91.6216) (44.8542, -91.5033) (45.2247, -91.2306) (45.3687, -91.1585) knots 0 0 0 1 2 2 2
  spline S71 degree 2 poles (45.3687, -91.1585) (45.5437, -91.0762) (45.8936, -90.9887) (46.1355, -90.9887) knots 0 0 0 1 2 2 2
  spline S72 degree 2 poles (46.1355, -90.9887) (46.9537, -90.9887) (47.9108, -92.3472) (47.9108, -93.4793) knots 0 0 0 1 2 2 2
  spline S73 degree 2 poles (47.9108, -93.4793) (47.9108, -94.1071) (47.5866, -95.0282) (47.3036, -95.3678) knots 0 0 0 1 2 2 2
  spline S74 degree 2 poles (47.3036, -95.3678) (47.0411, -95.6817) (46.3001, -96.0419) (45.8885, -96.0419) knots 0 0 0 1 2 2 2
  spline S75 degree 2 poles (45.8885, -96.0419) (45.5128, -96.0419) (45.0291, -95.8824) (44.7101, -95.7178) knots 0 0 0 1 2 2 2
  line L48 (44.7101, -95.7178) -> (44.7101, -97.7555)
  line L49 (44.7101, -97.7555) -> (43.2178, -97.7555)
  line L50 (43.2178, -97.7555) -> (43.2178, -91.1225)
  line L51 (44.7101, -92.4398) -> (44.7101, -94.7915)
  spline S76 degree 2 poles (44.7101, -94.7915) (44.8181, -94.8481) (45.1783, -94.9201) (45.307, -94.9201) knots 0 0 0 1 2 2 2
  spline S77 degree 2 poles (45.307, -94.9201) (45.8422, -94.9201) (46.3825, -94.1689) (46.3825, -93.4947) knots 0 0 0 1 2 2 2
  spline S78 degree 2 poles (46.3825, -93.4947) (46.3825, -92.7846) (45.9502, -92.1517) (45.4717, -92.1517) knots 0 0 0 1 2 2 2
  spline S79 degree 2 poles (45.4717, -92.1517) (45.2761, -92.1517) (44.8747, -92.306) (44.7101, -92.4398) knots 0 0 0 1 2 2 2
  spline S80 degree 2 poles (34.8249, -93.5822) (34.8249, -92.4398) (35.9827, -91.0299) (36.842, -91.0299) knots 0 0 0 1 2 2 2
  spline S81 degree 2 poles (36.842, -91.0299) (37.1971, -91.0299) (37.7271, -91.1894) (38.0256, -91.3592) knots 0 0 0 1 2 2 2
  line L52 (38.0256, -91.3592) -> (38.0873, -91.1225)
  line L53 (38.0873, -91.1225) -> (39.5179, -91.1225)
  line L54 (39.5179, -91.1225) -> (39.5179, -97.7555)
  line L55 (39.5179, -97.7555) -> (38.0256, -97.7555)
  line L56 (38.0256, -97.7555) -> (38.0256, -95.409)
  spline S82 degree 2 poles (38.0256, -95.409) (37.6963, -95.692) (37.017, -96.0419) (36.5693, -96.0419) knots 0 0 0 1 2 2 2
  spline S83 degree 2 poles (36.5693, -96.0419) (35.7305, -96.0419) (34.8249, -94.74) (34.8249, -93.5822) knots 0 0 0 1 2 2 2
  spline S84 degree 2 poles (36.3532, -93.5513) (36.3532, -94.2666) (36.7854, -94.879) (37.2383, -94.879) knots 0 0 0 1 2 2 2
  spline S85 degree 2 poles (37.2383, -94.879) (37.439, -94.879) (37.8352, -94.7503) (38.0256, -94.6217) knots 0 0 0 1 2 2 2
  line L57 (38.0256, -94.6217) -> (38.0256, -92.2237)
  spline S86 degree 2 poles (38.0256, -92.2237) (37.8764, -92.162) (37.5728, -92.1208) (37.4235, -92.1208) knots 0 0 0 1 2 2 2
  spline S87 degree 2 poles (37.4235, -92.1208) (36.8832, -92.1208) (36.3532, -92.8361) (36.3532, -93.5513) knots 0 0 0 1 2 2 2
  line L58 (29.5349, -95.9133) -> (31.9483, -89.3678)
  line L59 (31.9483, -89.3678) -> (33.5538, -89.3678)
  line L60 (33.5538, -89.3678) -> (32.8283, -91.2409)
  line L61 (32.8283, -91.2409) -> (34.583, -95.9133)
  line L62 (34.583, -95.9133) -> (33.0187, -95.9133)
  line L63 (33.0187, -95.9133) -> (32.0101, -92.9081)
  line L64 (32.0101, -92.9081) -> (31.0684, -95.9133)
  line L65 (31.0684, -95.9133) -> (29.5349, -95.9133)
  line L66 (73.4858, -80.4871) -> (75.4257, -80.4871)
  line L67 (75.4257, -80.4871) -> (77.1908, -82.8182)
  line L68 (77.1908, -82.8182) -> (77.7671, -82.8182)
  line L69 (77.7671, -82.8182) -> (77.7671, -80.4871)
  line L70 (77.7671, -80.4871) -> (79.352, -80.4871)
  line L71 (79.352, -80.4871) -> (79.352, -86.8371)
  line L72 (79.352, -86.8371) -> (76.7997, -86.8371)
  spline S88 degree 2 poles (76.7997, -86.8371) (76.2697, -86.8371) (75.4875, -86.7033) (75.153, -86.4975) knots 0 0 0 1 2 2 2
  spline S89 degree 2 poles (75.153, -86.4975) (74.8134, -86.2814) (74.412, -85.6073) (74.412, -85.0927) knots 0 0 0 1 2 2 2
  spline S90 degree 2 poles (74.412, -85.0927) (74.412, -84.3671) (75.0707, -83.4563) (75.6213, -83.1887) knots 0 0 0 1 2 2 2
  line L73 (75.6213, -83.1887) -> (73.4858, -80.4871)
  spline S91 degree 2 poles (76.0484, -84.892) (76.0484, -85.1339) (76.2337, -85.4786) (76.4446, -85.5713) knots 0 0 0 1 2 2 2
  spline S92 degree 2 poles (76.4446, -85.5713) (76.5939, -85.633) (76.9592, -85.669) (77.2319, -85.669) knots 0 0 0 1 2 2 2
  line L74 (77.2319, -85.669) -> (77.7671, -85.669)
  line L75 (77.7671, -85.669) -> (77.7671, -83.9606)
  line L76 (77.7671, -83.9606) -> (77.3091, -83.9606)
  spline S93 degree 2 poles (77.3091, -83.9606) (76.9798, -83.9606) (76.5115, -84.0429) (76.352, -84.1716) knots 0 0 0 1 2 2 2
  spline S94 degree 2 poles (76.352, -84.1716) (76.1976, -84.2951) (76.0484, -84.6244) (76.0484, -84.892) knots 0 0 0 1 2 2 2
  spline S95 degree 2 poles (68.5046, -82.88) (68.5046, -81.6964) (69.7962, -80.3379) (70.9746, -80.3379) knots 0 0 0 1 2 2 2
  spline S96 degree 2 poles (70.9746, -80.3379) (72.1478, -80.3379) (73.4497, -81.6964) (73.4497, -82.88) knots 0 0 0 1 2 2 2
  spline S97 degree 2 poles (73.4497, -82.88) (73.4497, -84.0738) (72.1478, -85.4272) (70.9746, -85.4272) knots 0 0 0 1 2 2 2
  spline S98 degree 2 poles (70.9746, -85.4272) (69.8013, -85.4272) (68.5046, -84.0687) (68.5046, -82.88) knots 0 0 0 1 2 2 2
  spline S99 degree 2 poles (70.0329, -82.8697) (70.0329, -83.2968) (70.1718, -83.868) (70.2953, -84.0378) knots 0 0 0 1 2 2 2
  spline S100 degree 2 poles (70.2953, -84.0378) (70.4291, -84.2179) (70.7636, -84.3568) (70.9746, -84.3568) knots 0 0 0 1 2 2 2
  spline S101 degree 2 poles (70.9746, -84.3568) (71.1804, -84.3568) (71.5046, -84.2333) (71.6384, -84.0584) knots 0 0 0 1 2 2 2
  spline S102 degree 2 poles (71.6384, -84.0584) (71.767, -83.8937) (71.9214, -83.3122) (71.9214, -82.8697) knots 0 0 0 1 2 2 2
  spline S103 degree 2 poles (71.9214, -82.8697) (71.9214, -82.4323) (71.7773, -81.892) (71.659, -81.7273) knots 0 0 0 1 2 2 2
  spline S104 degree 2 poles (71.659, -81.7273) (71.5406, -81.5626) (71.1804, -81.4082) (70.9643, -81.4082) knots 0 0 0 1 2 2 2
  spline S105 degree 2 poles (70.9643, -81.4082) (70.7842, -81.4082) (70.4137, -81.5626) (70.3005, -81.717) knots 0 0 0 1 2 2 2
  spline S106 degree 2 poles (70.3005, -81.717) (70.1718, -81.8971) (70.0329, -82.4168) (70.0329, -82.8697) knots 0 0 0 1 2 2 2
  spline S107 degree 2 poles (63.0191, -82.9469) (63.0191, -81.8045) (64.1769, -80.3945) (65.0362, -80.3945) knots 0 0 0 1 2 2 2
  spline S108 degree 2 poles (65.0362, -80.3945) (65.3913, -80.3945) (65.9213, -80.554) (66.2198, -80.7238) knots 0 0 0 1 2 2 2
  line L77 (66.2198, -80.7238) -> (66.2815, -80.4871)
  line L78 (66.2815, -80.4871) -> (67.7121, -80.4871)
  line L79 (67.7121, -80.4871) -> (67.7121, -87.1202)
  line L80 (67.7121, -87.1202) -> (66.2198, -87.1202)
  line L81 (66.2198, -87.1202) -> (66.2198, -84.7736)
  spline S109 degree 2 poles (66.2198, -84.7736) (65.8905, -85.0567) (65.2112, -85.4066) (64.7635, -85.4066) knots 0 0 0 1 2 2 2
  spline S110 degree 2 poles (64.7635, -85.4066) (63.9247, -85.4066) (63.0191, -84.1047) (63.0191, -82.9469) knots 0 0 0 1 2 2 2
  spline S111 degree 2 poles (64.5474, -82.916) (64.5474, -83.6313) (64.9796, -84.2436) (65.4325, -84.2436) knots 0 0 0 1 2 2 2
  spline S112 degree 2 poles (65.4325, -84.2436) (65.6332, -84.2436) (66.0294, -84.115) (66.2198, -83.9863) knots 0 0 0 1 2 2 2
  line L82 (66.2198, -83.9863) -> (66.2198, -81.5884)
  spline S113 degree 2 poles (66.2198, -81.5884) (66.0706, -81.5266) (65.767, -81.4854) (65.6177, -81.4854) knots 0 0 0 1 2 2 2
  spline S114 degree 2 poles (65.6177, -81.4854) (65.0774, -81.4854) (64.5474, -82.2007) (64.5474, -82.916) knots 0 0 0 1 2 2 2
  spline S115 degree 2 poles (57.5902, -80.3739) (58.3209, -80.3739) (59.4221, -80.657) (59.8955, -80.8628) knots 0 0 0 1 2 2 2
  line L83 (59.8955, -80.8628) -> (59.8955, -82.3757)
  line L84 (59.8955, -82.3757) -> (59.7514, -82.3757)
  spline S116 degree 2 poles (59.7514, -82.3757) (59.2729, -81.9691) (58.1253, -81.5317) (57.585, -81.5317) knots 0 0 0 1 2 2 2
  spline S117 degree 2 poles (57.585, -81.5317) (57.4461, -81.5317) (56.9984, -81.5935) (56.8646, -81.6553) knots 0 0 0 1 2 2 2
  spline S118 degree 2 poles (56.8646, -81.6553) (56.6999, -81.7273) (56.4684, -81.9897) (56.4684, -82.2007) knots 0 0 0 1 2 2 2
  spline S119 degree 2 poles (56.4684, -82.2007) (56.4684, -82.4426) (56.844, -82.741) (57.1013, -82.8079) knots 0 0 0 1 2 2 2
  spline S120 degree 2 poles (57.1013, -82.8079) (57.4255, -82.8954) (58.1614, -83.0446) (58.4856, -83.1578) knots 0 0 0 1 2 2 2
  spline S121 degree 2 poles (58.4856, -83.1578) (59.2214, -83.4151) (59.8595, -84.2951) (59.8595, -84.9538) knots 0 0 0 1 2 2 2
  spline S122 degree 2 poles (59.8595, -84.9538) (59.8595, -85.844) (58.3518, -86.9503) (57.2197, -86.9503) knots 0 0 0 1 2 2 2
  spline S123 degree 2 poles (57.2197, -86.9503) (56.6536, -86.9503) (55.5318, -86.7188) (55.0893, -86.5232) knots 0 0 0 1 2 2 2
  line L85 (55.0893, -86.5232) -> (55.0893, -85.0721)
  line L86 (55.0893, -85.0721) -> (55.2282, -85.0721)
  spline S124 degree 2 poles (55.2282, -85.0721) (55.5833, -85.3757) (56.6022, -85.7925) (57.1373, -85.7925) knots 0 0 0 1 2 2 2
  spline S125 degree 2 poles (57.1373, -85.7925) (57.3483, -85.7925) (57.6777, -85.7308) (57.8629, -85.6484) knots 0 0 0 1 2 2 2
  spline S126 degree 2 poles (57.8629, -85.6484) (58.0121, -85.5815) (58.2283, -85.314) (58.2283, -85.1493) knots 0 0 0 1 2 2 2
  spline S127 degree 2 poles (58.2283, -85.1493) (58.2283, -84.9023) (57.8835, -84.6193) (57.3895, -84.5061) knots 0 0 0 1 2 2 2
  spline S128 degree 2 poles (57.3895, -84.5061) (57.0704, -84.434) (56.4787, -84.2951) (56.139, -84.1767) knots 0 0 0 1 2 2 2
  spline S129 degree 2 poles (56.139, -84.1767) (55.4804, -83.9349) (54.8371, -83.1321) (54.8371, -82.4734) knots 0 0 0 1 2 2 2
  spline S130 degree 2 poles (54.8371, -82.4734) (54.8371, -81.5266) (56.3243, -80.3739) (57.5902, -80.3739) knots 0 0 0 1 2 2 2
  spline S131 degree 2 poles (52.2745, -80.3945) (53.1853, -80.3945) (54.0189, -81.1458) (54.0189, -82) knots 0 0 0 1 2 2 2
  line L87 (54.0189, -82) -> (54.0189, -84.2385)
  line L88 (54.0189, -84.2385) -> (54.5901, -84.2385)
  line L89 (54.5901, -84.2385) -> (54.5901, -85.2779)
  line L90 (54.5901, -85.2779) -> (54.0189, -85.2779)
  line L91 (54.0189, -85.2779) -> (54.0189, -86.6467)
  line L92 (54.0189, -86.6467) -> (52.5266, -86.6467)
  line L93 (52.5266, -86.6467) -> (52.5266, -85.2779)
  line L94 (52.5266, -85.2779) -> (51.0858, -85.2779)
  line L95 (51.0858, -85.2779) -> (51.0858, -84.2385)
  line L96 (51.0858, -84.2385) -> (52.5266, -84.2385)
  line L97 (52.5266, -84.2385) -> (52.5266, -82.5352)
  spline S132 degree 2 poles (52.5266, -82.5352) (52.5266, -82.283) (52.5164, -81.9074) (52.4546, -81.7582) knots 0 0 0 1 2 2 2
  spline S133 degree 2 poles (52.4546, -81.7582) (52.3928, -81.6089) (52.0892, -81.434) (51.8011, -81.434) knots 0 0 0 1 2 2 2
  spline S134 degree 2 poles (51.8011, -81.434) (51.6776, -81.434) (51.2916, -81.5369) (51.2144, -81.5781) knots 0 0 0 1 2 2 2
  line L98 (51.2144, -81.5781) -> (51.0858, -81.5781)
  line L99 (51.0858, -81.5781) -> (51.0858, -80.5283)
  spline S135 degree 2 poles (51.0858, -80.5283) (51.3277, -80.4666) (51.8731, -80.3945) (52.2745, -80.3945) knots 0 0 0 1 2 2 2
  spline S136 degree 2 poles (48.024, -80.3585) (49.3825, -80.3585) (50.8285, -81.6553) (50.8285, -82.8542) knots 0 0 0 1 2 2 2
  spline S137 degree 2 poles (50.8285, -82.8542) (50.8285, -84.0275) (49.4803, -85.4272) (48.2659, -85.4272) knots 0 0 0 1 2 2 2
  spline S138 degree 2 poles (48.2659, -85.4272) (47.1698, -85.4272) (46.0583, -84.2385) (46.0583, -83.1373) knots 0 0 0 1 2 2 2
  line L100 (46.0583, -83.1373) -> (46.0583, -82.5969)
  line L101 (46.0583, -82.5969) -> (49.3362, -82.5969)
  spline S139 degree 2 poles (49.3362, -82.5969) (49.3156, -82.2625) (49.0738, -81.8199) (48.8782, -81.6861) knots 0 0 0 1 2 2 2
  spline S140 degree 2 poles (48.8782, -81.6861) (48.6878, -81.5523) (48.1732, -81.4391) (47.8696, -81.4391) knots 0 0 0 1 2 2 2
  spline S141 degree 2 poles (47.8696, -81.4391) (47.6123, -81.4391) (47.108, -81.5523) (46.8971, -81.6501) knots 0 0 0 1 2 2 2
  spline S142 degree 2 poles (46.8971, -81.6501) (46.7118, -81.7273) (46.4031, -81.9177) (46.3053, -81.9897) knots 0 0 0 1 2 2 2
  line L102 (46.3053, -81.9897) -> (46.1458, -81.9897)
  line L103 (46.1458, -81.9897) -> (46.1458, -80.7547)
  spline S143 degree 2 poles (46.1458, -80.7547) (46.331, -80.6827) (46.6295, -80.5592) (46.8971, -80.4974) knots 0 0 0 1 2 2 2
  spline S144 degree 2 poles (46.8971, -80.4974) (47.1389, -80.4305) (47.6535, -80.3585) (48.024, -80.3585) knots 0 0 0 1 2 2 2
  spline S145 degree 2 poles (47.53, -83.4975) (47.5403, -83.9709) (47.9571, -84.47) (48.3842, -84.47) knots 0 0 0 1 2 2 2
  spline S146 degree 2 poles (48.3842, -84.47) (48.8216, -84.47) (49.3156, -83.9452) (49.3414, -83.4975) knots 0 0 0 1 2 2 2
  line L104 (49.3414, -83.4975) -> (47.53, -83.4975)
  spline S147 degree 2 poles (42.837, -80.3585) (44.1955, -80.3585) (45.6415, -81.6553) (45.6415, -82.8542) knots 0 0 0 1 2 2 2
  spline S148 degree 2 poles (45.6415, -82.8542) (45.6415, -84.0275) (44.2933, -85.4272) (43.0788, -85.4272) knots 0 0 0 1 2 2 2
  spline S149 degree 2 poles (43.0788, -85.4272) (41.9828, -85.4272) (40.8713, -84.2385) (40.8713, -83.1373) knots 0 0 0 1 2 2 2
  line L105 (40.8713, -83.1373) -> (40.8713, -82.5969)
  line L106 (40.8713, -82.5969) -> (44.1492, -82.5969)
  spline S150 degree 2 poles (44.1492, -82.5969) (44.1286, -82.2625) (43.8867, -81.8199) (43.6912, -81.6861) knots 0 0 0 1 2 2 2
  spline S151 degree 2 poles (43.6912, -81.6861) (43.5008, -81.5523) (42.9862, -81.4391) (42.6826, -81.4391) knots 0 0 0 1 2 2 2
  spline S152 degree 2 poles (42.6826, -81.4391) (42.4253, -81.4391) (41.921, -81.5523) (41.71, -81.6501) knots 0 0 0 1 2 2 2
  spline S153 degree 2 poles (41.71, -81.6501) (41.5248, -81.7273) (41.216, -81.9177) (41.1183, -81.9897) knots 0 0 0 1 2 2 2
  line L107 (41.1183, -81.9897) -> (40.9587, -81.9897)
  line L108 (40.9587, -81.9897) -> (40.9587, -80.7547)
  spline S154 degree 2 poles (40.9587, -80.7547) (41.144, -80.6827) (41.4424, -80.5592) (41.71, -80.4974) knots 0 0 0 1 2 2 2
  spline S155 degree 2 poles (41.71, -80.4974) (41.9519, -80.4305) (42.4665, -80.3585) (42.837, -80.3585) knots 0 0 0 1 2 2 2
  spline S156 degree 2 poles (42.343, -83.4975) (42.3533, -83.9709) (42.7701, -84.47) (43.1972, -84.47) knots 0 0 0 1 2 2 2
  spline S157 degree 2 poles (43.1972, -84.47) (43.6346, -84.47) (44.1286, -83.9452) (44.1543, -83.4975) knots 0 0 0 1 2 2 2
  line L109 (44.1543, -83.4975) -> (42.343, -83.4975)
  line L110 (38.6122, -80.4871) -> (40.1045, -80.4871)
  line L111 (40.1045, -80.4871) -> (40.1045, -87.1202)
  line L112 (40.1045, -87.1202) -> (38.6122, -87.1202)
  line L113 (38.6122, -87.1202) -> (38.6122, -80.4871)